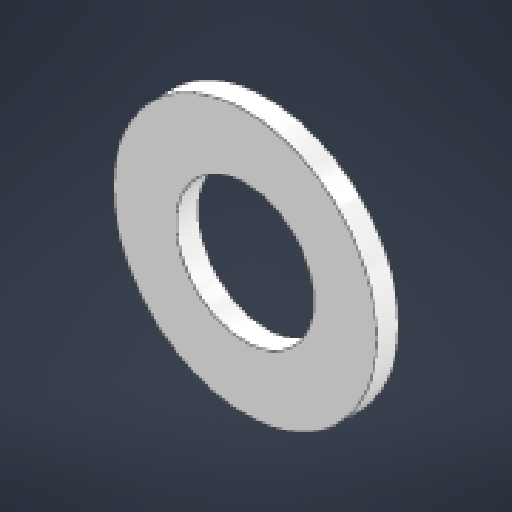
# Autodesk Inventor part: TT-0612-101
Saved by Autodesk Inventor 2024.3 (Build 283343000, 343)
## iProperties
Part Number: TT-0612-101
Material: 열가소성 수지
Catalog Web Link: https://www.hirosugi-net.co.jp/shop/g/g31822/
Description: ReadyMade
Document SubType Name: Sheet Metal
Designer: ASUS
Mass: 0.16644 g
Surface Area: 2.21341 cm^2
Volume: 0.0819249 cm^3
Density: 1.28 g/cm^3
Sheet Metal Rule: 기본값
Appearance: 滑らか - 白
Author: Masato Kubotera
Autodesk Inventor part; units mm, degrees
ref_plane "YZ Plane" through (0, 0, 0) normal (1, 0, 0) x (0, 1, 0)
ref_plane "XZ Plane" through (0, 0, 0) normal (0, 1, 0) x (-1, 0, 0)
ref_plane "XY Plane" through (0, 0, 0) normal (0, 0, 1) x (1, 0, 0)
sketch "スケッチ1" plane through (0, 0, 0) normal (0, 0, 1) x (1, 0, 0)
  circle A0 centre (0, 0) radius 3.125
  circle A1 centre (0, 0) radius 6
  dimension "d0" = 6.25
  dimension "d1" = 12
  constraints: 2 centre point, 2 coincident
  measures "d0" diameter of A0
  measures "d1" diameter of A1
extrude "押し出し1" add sketch "スケッチ1" along normal blind 1
equation "\"TransitionRadius\" = BendRadius"
equation "\"BendRadius\" = 3.048"
